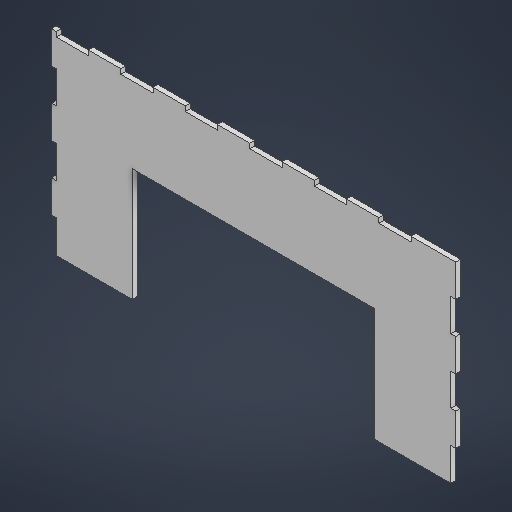
# Autodesk Inventor part: Part1
Saved by Autodesk Inventor 2027.1 (Build 311270010, 270A)
## iProperties
Created: 2026-10-07
Part Number: Part1
Material: Generic
Document SubType Name: Modeling
Designer: daniel
Density: 1 g/cm^3
Appearance: Default
Author: daniel
Autodesk Inventor part; units mm, degrees
ref_plane "YZ Plane" through (0, 0, 0) normal (1, 0, 0) x (0, 1, 0)
ref_plane "XZ Plane" through (0, 0, 0) normal (0, 1, 0) x (-1, 0, 0)
ref_plane "XY Plane" through (0, 0, 0) normal (0, 0, 1) x (1, 0, 0)
sketch "Sketch1" plane through (0, 0, 0) normal (0, 0, 1) x (1, 0, 0)
  line L0 (-37.6936, 53.8926) -> (212.3064, 53.8926)
  line L1 (212.3064, 53.8926) -> (212.3064, -66.1074)
  line L2 (212.3064, -66.1074) -> (-37.6936, -66.1074)
  line L3 (-37.6936, -66.1074) -> (-37.6936, 53.8926)
  line L4 (12.3064, -66.1074) -> (162.3064, -66.1074)
  line L5 (162.3064, -66.1074) -> (162.3064, 3.8926)
  line L6 (162.3064, 3.8926) -> (12.3064, 3.8926)
  line L7 (12.3064, 3.8926) -> (12.3064, -66.1074)
  line L8 (-37.6936, 53.8926) -> (-34.6936, 53.8926)
  line L9 (-34.6936, 53.8926) -> (-34.6936, 33.8926)
  line L10 (-34.6936, 33.8926) -> (-37.6936, 33.8926)
  line L11 (-37.6936, 33.8926) -> (-37.6936, 53.8926)
  line L12 (-37.6936, 33.8926) -> (-34.6936, 33.8926)
  line L13 (-34.6936, 33.8926) -> (-34.6936, 13.9926)
  line L14 (-34.6936, 13.9926) -> (-37.6936, 13.9926)
  line L15 (-37.6936, 13.9926) -> (-37.6936, 33.8926)
  line L16 (-37.6936, 13.9926) -> (-34.6936, 13.9926)
  line L17 (-34.6936, 13.9926) -> (-34.6936, -6.0074)
  line L18 (-34.6936, -6.0074) -> (-37.6936, -6.0074)
  line L19 (-37.6936, -6.0074) -> (-37.6936, 13.9926)
  line L20 (-34.6936, -6.0074) -> (-37.6936, -6.0074)
  line L21 (-37.6936, -6.0074) -> (-37.6936, -25.9074)
  line L22 (-37.6936, -25.9074) -> (-34.6936, -25.9074)
  line L23 (-34.6936, -25.9074) -> (-34.6936, -6.0074)
  line L24 (-37.6936, -25.9074) -> (-34.6936, -25.9074)
  line L25 (-34.6936, -25.9074) -> (-34.6936, -45.9074)
  line L26 (-34.6936, -45.9074) -> (-37.6936, -45.9074)
  line L27 (-37.6936, -45.9074) -> (-37.6936, -25.9074)
  line L28 (-34.6936, -45.9074) -> (-37.6936, -45.9074)
  line L29 (-37.6936, -45.9074) -> (-37.6936, -66.1074)
  line L30 (-37.6936, -66.1074) -> (-34.6936, -66.1074)
  line L31 (-34.6936, -66.1074) -> (-34.6936, -45.9074)
  line L32 (212.3064, -66.1074) -> (212.3064, 53.8926)
  line L33 (212.3064, 53.8926) -> (209.3064, 53.8926)
  line L34 (209.3064, 53.8926) -> (209.3064, 33.8926)
  line L35 (209.3064, 33.8926) -> (212.3064, 33.8926)
  line L36 (212.3064, 33.8926) -> (212.3064, 53.8926)
  line L37 (212.3064, 33.8926) -> (209.3064, 33.8926)
  line L38 (209.3064, 33.8926) -> (209.3064, 13.9926)
  line L39 (209.3064, 13.9926) -> (212.3064, 13.9926)
  line L40 (212.3064, 13.9926) -> (212.3064, 33.8926)
  line L41 (212.3064, 13.9926) -> (209.3064, 13.9926)
  line L42 (209.3064, 13.9926) -> (209.3064, -6.0074)
  line L43 (209.3064, -6.0074) -> (212.3064, -6.0074)
  line L44 (212.3064, -6.0074) -> (212.3064, 13.9926)
  line L45 (209.3064, -6.0074) -> (212.3064, -6.0074)
  line L46 (212.3064, -6.0074) -> (212.3064, -25.9074)
  line L47 (212.3064, -25.9074) -> (209.3064, -25.9074)
  line L48 (209.3064, -25.9074) -> (209.3064, -6.0074)
  line L49 (212.3064, -25.9074) -> (209.3064, -25.9074)
  line L50 (209.3064, -25.9074) -> (209.3064, -45.9074)
  line L51 (209.3064, -45.9074) -> (212.3064, -45.9074)
  line L52 (212.3064, -45.9074) -> (212.3064, -25.9074)
  line L53 (209.3064, -45.9074) -> (212.3064, -45.9074)
  line L54 (212.3064, -45.9074) -> (212.3064, -66.1074)
  line L55 (212.3064, -66.1074) -> (209.3064, -66.1074)
  line L56 (209.3064, -66.1074) -> (209.3064, -45.9074)
  line L57 (-34.6936, 53.8926) -> (-14.7936, 53.8926)
  line L58 (-14.7936, 53.8926) -> (-14.7936, 50.8926)
  line L59 (-14.7936, 50.8926) -> (-34.6936, 50.8926)
  line L60 (-34.6936, 50.8926) -> (-34.6936, 53.8926)
  line L61 (-14.7936, 50.8926) -> (5.2064, 50.8926)
  line L62 (5.2064, 50.8926) -> (5.2064, 53.8926)
  line L63 (5.2064, 53.8926) -> (-14.7936, 53.8926)
  line L64 (-14.7936, 53.8926) -> (-14.7936, 50.8926)
  line L65 (5.2064, 50.8926) -> (25.1064, 50.8926)
  line L66 (25.1064, 50.8926) -> (25.1064, 53.8926)
  line L67 (25.1064, 53.8926) -> (5.2064, 53.8926)
  line L68 (5.2064, 53.8926) -> (5.2064, 50.8926)
  line L69 (25.1064, 50.8926) -> (45.1064, 50.8926)
  line L70 (45.1064, 50.8926) -> (45.1064, 53.8926)
  line L71 (45.1064, 53.8926) -> (25.1064, 53.8926)
  line L72 (25.1064, 53.8926) -> (25.1064, 50.8926)
  line L73 (45.1064, 50.8926) -> (65.0064, 50.8926)
  line L74 (65.0064, 50.8926) -> (65.0064, 53.8926)
  line L75 (65.0064, 53.8926) -> (45.1064, 53.8926)
  line L76 (45.1064, 53.8926) -> (45.1064, 50.8926)
  line L77 (65.0064, 50.8926) -> (85.0064, 50.8926)
  line L78 (85.0064, 50.8926) -> (85.0064, 53.8926)
  line L79 (85.0064, 53.8926) -> (65.0064, 53.8926)
  line L80 (65.0064, 53.8926) -> (65.0064, 50.8926)
  line L81 (85.0064, 50.8926) -> (104.9064, 50.8926)
  line L82 (104.9064, 50.8926) -> (104.9064, 53.8926)
  line L83 (104.9064, 53.8926) -> (85.0064, 53.8926)
  line L84 (85.0064, 53.8926) -> (85.0064, 50.8926)
  line L85 (104.9064, 50.8926) -> (124.9064, 50.8926)
  line L86 (124.9064, 50.8926) -> (124.9064, 53.8926)
  line L87 (124.9064, 53.8926) -> (104.9064, 53.8926)
  line L88 (104.9064, 53.8926) -> (104.9064, 50.8926)
  line L89 (124.9064, 50.8926) -> (144.8064, 50.8926)
  line L90 (144.8064, 50.8926) -> (144.8064, 53.8926)
  line L91 (144.8064, 53.8926) -> (124.9064, 53.8926)
  line L92 (124.9064, 53.8926) -> (124.9064, 50.8926)
  line L93 (144.8064, 50.8926) -> (164.8064, 50.8926)
  line L94 (164.8064, 50.8926) -> (164.8064, 53.8926)
  line L95 (164.8064, 53.8926) -> (144.8064, 53.8926)
  line L96 (144.8064, 53.8926) -> (144.8064, 50.8926)
  line L97 (164.8064, 50.8926) -> (184.7064, 50.8926)
  line L98 (184.7064, 50.8926) -> (184.7064, 53.8926)
  line L99 (184.7064, 53.8926) -> (164.8064, 53.8926)
  line L100 (164.8064, 53.8926) -> (164.8064, 50.8926)
  line L101 (184.7064, 50.8926) -> (209.3064, 50.8926)
  line L102 (209.3064, 50.8926) -> (209.3064, 53.8926)
  line L103 (209.3064, 53.8926) -> (184.7064, 53.8926)
  line L104 (184.7064, 53.8926) -> (184.7064, 50.8926)
  point P0 (0, 0)
  point P1 (212.3064, -45.9074)
  point P2 (212.3064, -25.9074)
  point P3 (212.3064, -6.0074)
  point P4 (212.3064, 13.9926)
  point P5 (212.3064, 33.8926)
  point P6 (-37.6936, 13.9926)
  point P7 (-14.7936, 53.8926)
  point P8 (-34.6936, 50.8926)
  point P9 (209.3064, 53.8926)
  point P10 (212.3064, 13.9926)
  point P11 (212.3064, 23.9426)
  point P12 (209.3064, 23.9426)
  point P13 (212.3064, -15.9574)
  point P14 (209.3064, -15.9574)
  dimension "d0" = 250
  dimension "d1" = 120
  dimension "d14" = 150
  dimension "d15" = 70
  dimension "d16" = 50
  dimension "d17" = 3
  dimension "d18" = 20
  dimension "d19" = 19.9
  dimension "d20" = 20
  dimension "d21" = 19.9
  dimension "d22" = 20
  dimension "d25" = 19.9
  dimension "d26" = 3
  dimension "d27" = 20
  dimension "d28" = 19.9
  dimension "d29" = 20
  dimension "d30" = 19.9
  dimension "d31" = 20
  dimension "d32" = 19.9
  dimension "d33" = 20
  dimension "d34" = 19.9
  dimension "d35" = 20
  dimension "d36" = 19.9
  dimension "d37" = 3
  dimension "d38" = 3
  constraints: 208 end point, 39 parallel, 20 horizontal, 19 perpendicular, 9 point on line, 4 midpoint, 1 vertical, 13 other
  measures "d0" distance of L1.end L2.end
  measures "d1" distance of L1.start L1.end
  measures "d14" distance of L6.end L5.end
  measures "d15" distance of L5.end L4.end
  measures "d16" distance between parallel lines of L1 L5
  measures "d17" distance of L9.end L10.end
  measures "d18" distance of L8.end L9.end
  measures "d19" distance of L12.end L13.end
  measures "d20" distance of L16.end L17.end
  measures "d21" distance of L21.end L20.end
  measures "d22" distance of L24.end L25.end
  measures "d25" distance of L58.end L59.end
  measures "d26" distance of L57.end L58.end
  measures "d27" distance of L63.end L62.end
  measures "d28" distance of L67.end L66.end
  measures "d29" distance of L71.end L70.end
  measures "d30" distance of L75.end L74.end
  measures "d31" distance of L79.end L78.end
  measures "d32" distance of L83.end L82.end
  measures "d33" distance of L87.end L86.end
  measures "d34" distance of L91.end L90.end
  measures "d35" distance of L95.end L94.end
  measures "d36" distance of L99.end L98.end
  measures "d37" distance of point (212.306, 23.943) point (209.306, 23.943)
  measures "d38" distance of point (212.306, -15.957) point (209.306, -15.957)
extrude "Extrusion1" add sketch "Sketch1" along normal blind 3 contours L0 L9 L10 L3 | L0 L62 L61 L58 | L59 L61 L65 L69 L73 L77 L81 L85 L89 L93 L97 L101 L34 L38 L42 L48 L50 L56 L2 L5 L6 L7 L31 L25 L23 L17 L13 L9 | L14 L17 L18 L3 | L0 L70 L69 L66 | L22 L25 L26 L3 | L0 L78 L77 L74 | L0 L86 L85 L82 | L0 L94 L93 L90 | L50 L47 L1 L51 | L0 L34 L101 L98 | L0 L1 L35 L34 | L42 L39 L1 L43
equation "\"d16\" = -0.5 * d14 + 0.5 * d0"
equation "\"d19\" = d25"
equation "\"d21\" = d25"
equation "\"d28\" = d25"
equation "\"d30\" = d25"
body "Solid1"
